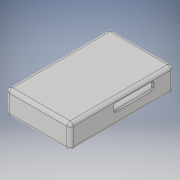
# Autodesk Inventor part: case
Saved by Autodesk Inventor 2019 (Build 230136000, 136)
## iProperties
Created: 2018-08-27
Part Number: case
Material: Generic
Document SubType Name: Modeling
Designer: ABiri-Mobile
Density: 1 g/cm^3
Appearance: Default
Author: ABiri-Mobile
Autodesk Inventor part; units mm, degrees
ref_plane "YZ Plane" through (0, 0, 0) normal (1, 0, 0) x (0, 1, 0)
ref_plane "XZ Plane" through (0, 0, 0) normal (0, 1, 0) x (-1, 0, 0)
ref_plane "XY Plane" through (0, 0, 0) normal (0, 0, 1) x (1, 0, 0)
sketch "Sketch4" plane through (0, 0, 0) normal (0, 1, 0) x (-1, 0, 0)
  line L0 (0, 0) -> (40, 0)
  line L1 (40, 0) -> (40, -65)
  line L2 (40, -65) -> (0, -65)
  line L3 (0, -65) -> (0, 0)
  dimension "d11" = 65
  dimension "d12" = 40
  constraints: 8 end point, 2 parallel, 1 horizontal, 1 perpendicular
  measures "d11" distance between parallel lines of L2 L0
  measures "d12" distance between parallel lines of L3 L1
extrude "Extrusion2" add sketch "Sketch4" along normal blind 15
fillet "Fillet3" radius 2 12 edges at (-20, 15, 0) (0, 15, -32.5) (0, 7.5, 0) (-40, 7.5, 0) (-20, 0, 0) (0, 0, -32.5) (0, 7.5, -65) (-20, 15, -65) (-40, 15, -32.5) (-20, 0, -65) (-40, 7.5, -65) (-40, 0, -32.5)
shell "Shell1" thickness 1.5 removed faces 0
sketch "Hole" plane through (0, 2, -2) normal (1, 0, 0) x (0, 0, -1)
  line L0 (26.5, 10.5) -> (49.5, 10.5)
  line L1 (50.5, 9.5) -> (50.5, 6.5)
  line L2 (49.5, 5.5) -> (26.5, 5.5)
  line L3 (25.5, 6.5) -> (25.5, 9.5)
  line L4 (63, 0) -> (63, 11) projected
  line L5 (61, 13) -> (0, 13) projected
  arc A0 (26.5, 10.5) -> (25.5, 9.5) centre (26.5, 9.5) ccw
  arc A1 (50.5, 9.5) -> (49.5, 10.5) centre (49.5, 9.5) ccw
  arc A2 (49.5, 5.5) -> (50.5, 6.5) centre (49.5, 6.5) ccw
  arc A3 (25.5, 6.5) -> (26.5, 5.5) centre (26.5, 6.5) ccw
  point P0 (-2, -2)
  dimension "d17" = 5
  dimension "d18" = 25
  dimension "d19" = 37.5
  dimension "d20" = 7.5
  dimension "d21" = 1
  constraints: 8 end point, 8 point on circle, 8 tangent, 4 centre point, 3 equal radius, 2 parallel, 1 horizontal, 1 perpendicular
  measures "d17" distance between parallel lines of L2 L0
  measures "d18" distance between parallel lines of L3 L1
  measures "d19" distance between parallel lines of L4 L3
  measures "d20" distance between parallel lines of L5 L2
  measures "d21" radius of A0
extrude "Extrusion3" cut sketch "Hole" against normal blind 15
body "Solid2"
